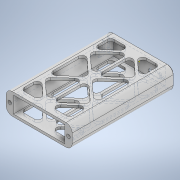
# Autodesk Inventor part: base
Saved by Autodesk Inventor 2021 (Build 250183000, 183)
## iProperties
Created: 2025-12-12
Part Number: base
Material: Generic
Document SubType Name: Modeling
Designer: Toby
Density: 1 g/cm^3
Appearance: Default
Author: Toby
Autodesk Inventor part; units mm, degrees
ref_plane "YZ Plane" through (0, 0, 0) normal (1, 0, 0) x (0, 1, 0)
ref_plane "XZ Plane" through (0, 0, 0) normal (0, 1, 0) x (-1, 0, 0)
ref_plane "XY Plane" through (0, 0, 0) normal (0, 0, 1) x (1, 0, 0)
sketch "Sketch1" plane through (0, 0, 0) normal (0, 0, 1) x (1, 0, 0)
  point P0 (0, 0)
sketch "Sketch2" plane through (0, 0, 0) normal (0, 0, 1) x (1, 0, 0)
  line L0 (-21, 6.75) -> (21, 6.75)
  line L1 (21, 6.75) -> (21, -6.75)
  line L2 (21, -6.75) -> (-21, -6.75)
  line L3 (-21, -6.75) -> (-21, 6.75)
  line L4 (-27, 8.75) -> (27, 8.75)
  line L5 (27, 8.75) -> (27, -8.75)
  line L6 (27, -8.75) -> (-27, -8.75)
  line L7 (-27, -8.75) -> (-27, 8.75)
  point P0 (0, 0)
  dimension "d0" = 42
  dimension "d1" = 13.5
  dimension "d2" = 2
  dimension "d3" = 2
  dimension "d4" = 6
  dimension "d5" = 6
  dimension "d6" = 6.75
  dimension "d7" = 21
  constraints: 16 end point, 4 parallel, 2 horizontal, 2 perpendicular
  measures "d0" distance of L0.start L0.end
  measures "d1" distance between parallel lines of L2 L0
  measures "d2" distance between parallel lines of L0 L4
  measures "d3" distance between parallel lines of L6 L2
  measures "d4" distance between parallel lines of L7 L3
  measures "d5" distance between parallel lines of L5 L1
  measures "d6" distance from line of point (0, 0) L0
  measures "d7" distance from line of point (0, 0) L3
extrude "Extrusion1" add sketch "Sketch2" along normal blind 82
sketch "Sketch3" plane through (0, 0, 0) normal (0, 0, -1) x (-1, 0, 0)
  line L0 (-27, -8.75) -> (-27, 8.75) projected
  line L1 (27, 8.75) -> (27, -8.75) projected
  line L2 (-27, 8.75) -> (27, 8.75)
  line L3 (27, 8.75) -> (27, -8.75)
  line L4 (27, -8.75) -> (-27, -8.75)
  line L5 (-27, -8.75) -> (-27, 8.75)
  point P0 (0, 0)
  constraints: 8 end point, 2 parallel, 1 horizontal, 1 perpendicular
extrude "Extrusion2" add sketch "Sketch3" along normal blind 1.2
fillet "Fillet1" radius 5 4 edges at (-27, 8.75, 40.4) (-27, -8.75, 40.4) (27, 8.75, 40.4) (27, -8.75, 40.4)
sketch "Sketch4" plane through (0, 0, 82) normal (0, 0, 1) x (1, 0, 0)
  line L0 (-21, -6.75) -> (-21, 6.75) projected
  line L1 (21, 6.75) -> (21, -6.75) projected
  line L2 (21, -6.75) -> (-21, -6.75) projected
  point P0 (0, 0)
  point P1 (-24, 0)
  point P2 (24, 0)
  dimension "d13" = 3
  dimension "d14" = 3
  dimension "d15" = 6.75
  dimension "d16" = 6.75
  measures "d13" distance from line of L0 point (-24, 0)
  measures "d14" distance from line of L1 point (24, 0)
  measures "d15" distance from line of L2 point (-24, 0)
  measures "d16" distance from line of L2 point (24, 0)
hole "Hole1" at (-24, 0, 82) at (24, 0, 82) direction (0, 0, -1) diameter 3 depth 8.8 tip angle 118
sketch "Sketch5" plane through (0, 0, 0) normal (0, 0, 1) x (1, 0, 0)
  line L0 (7.5, -1.05) -> (16.7, -1.05)
  line L1 (16.7, -1.05) -> (16.7, -4.55)
  line L2 (16.7, -4.55) -> (7.5, -4.55)
  line L3 (7.5, -4.55) -> (7.5, -1.05)
  line L4 (21, -6.75) -> (-21, -6.75) projected
  line L5 (21, 6.75) -> (21, -6.75) projected
  point P0 (0, 0)
  dimension "d24" = 2.2
  dimension "d25" = 3.5
  dimension "d26" = 9.2
  dimension "d27" = 4.3
  constraints: 8 end point, 2 parallel, 1 horizontal, 1 perpendicular
  measures "d24" distance between parallel lines of L4 L2
  measures "d25" distance between parallel lines of L2 L0
  measures "d26" distance of L0.start L0.end
  measures "d27" distance between parallel lines of L5 L1
extrude "Extrusion3" cut sketch "Sketch5" against normal blind 1.2
fillet "Fillet2" radius 1 4 edges at (16.7, -1.05, -0.6) (16.7, -4.55, -0.6) (7.5, -4.55, -0.6) (7.5, -1.05, -0.6)
sketch "Sketch6" plane through (0, 0, 0) normal (0, 0, 1) x (1, 0, 0)
  circle A0 centre (18.8, -2.8) radius 0.75
  line L0 (21, 6.75) -> (21, -6.75) projected
  line L1 (15.7, -4.55) -> (8.5, -4.55) projected
  line L2 (8.5, -1.05) -> (15.7, -1.05) projected
  point P0 (0, 0)
  dimension "d31" = 1.5
  dimension "d32" = 2.2
  dimension "d33" = 1.75
  dimension "d34" = 1.75
  constraints: 1 centre point
  measures "d31" diameter of A0
  measures "d32" distance from line of L0 A0.centre
  measures "d33" distance from line of L1 A0.centre
  measures "d34" distance from line of A0.centre L2
extrude "Extrusion4" cut sketch "Sketch6" against normal blind 1.2
chamfer "Chamfer1" distance 0.6 angle 45 8 edges at (12.1, -1.05, -1.2) (7.7929, -1.3429, -1.2) (7.5, -2.8, -1.2) (7.7929, -4.2571, -1.2) (12.1, -4.55, -1.2) (16.4071, -4.2571, -1.2) (16.7, -2.8, -1.2) (16.4071, -1.3429, -1.2)
chamfer "Chamfer2" distance 0.6 angle 45 8 edges at (0, 8.75, -1.2) (25.5355, 7.2855, -1.2) (27, 0, -1.2) (25.5355, -7.2855, -1.2) (0, -8.75, -1.2) (-25.5355, -7.2855, -1.2) (-27, 0, -1.2) (-25.5355, 7.2855, -1.2)
sketch "Sketch7" plane through (-22, 8.75, 82) normal (0, 1, 0) x (1, 0, 0)
  line L0 (2, 78.6) -> (42, 78.6)
  line L1 (42, 78.6) -> (42, 5)
  line L2 (42, 5) -> (2, 5)
  line L3 (2, 5) -> (2, 78.6)
  line L4 (0, 82.6) -> (44, 82.6) projected
  line L5 (0, 0) -> (0, 82.6) projected
  line L6 (44, 82.6) -> (44, 0) projected
  line L7 (44, 0) -> (0, 0) projected
  line L8 (44, 83.2) -> (48.4, 83.2) projected
  point P0 (22, 82)
  dimension "d43" = 4
  dimension "d44" = 2
  dimension "d45" = 2
  dimension "d46" = 5
  dimension "d47" = 4.6
  constraints: 8 end point, 2 parallel, 1 horizontal, 1 perpendicular
  measures "d43" distance between parallel lines of L0 L4
  measures "d44" distance between parallel lines of L5 L3
  measures "d45" distance between parallel lines of L6 L1
  measures "d46" distance between parallel lines of L7 L2
  measures "d47" distance between parallel lines of L0 L8
extrude "Extrusion5" cut sketch "Sketch7" against normal blind 30 contours L0 L1 L2 L3
sketch "Sketch8" plane through (-22, -8.75, 82) normal (0, -1, 0) x (1, 0, 0)
  line L0 (42, -5) -> (2, -5) projected
  line L1 (2, -78.6) -> (42, -78.6) projected
  line L2 (22, -5) -> (22, -78.6) construction
  line L3 (21, -5) -> (21, -78.6)
  line L4 (23, -78.6) -> (23, -5)
  arc A0 (23, -5) -> (21, -5) centre (22, -5) ccw
  arc A1 (21, -78.6) -> (23, -78.6) centre (22, -78.6) ccw
  line L5 (42, -78.6) -> (42, -5) projected
  line L6 (2, -5) -> (2, -78.6) projected
  line L7 (42, -23.4) -> (22, -5) construction
  line L8 (42.6771, -22.6641) -> (22.6771, -4.2641)
  line L9 (21.3229, -5.7359) -> (41.3229, -24.1359)
  arc A2 (41.3229, -24.1359) -> (42.6771, -22.6641) centre (42, -23.4) ccw
  arc A3 (22.6771, -4.2641) -> (21.3229, -5.7359) centre (22, -5) ccw
  line L10 (22, -5) -> (2, -23.4) construction
  line L11 (21.3229, -4.2641) -> (1.3229, -22.6641)
  line L12 (2.6771, -24.1359) -> (22.6771, -5.7359)
  arc A4 (22.6771, -5.7359) -> (21.3229, -4.2641) centre (22, -5) ccw
  arc A5 (1.3229, -22.6641) -> (2.6771, -24.1359) centre (2, -23.4) ccw
  line L13 (2, -23.4) -> (22, -41.8) construction
  arc A6 (2.6771, -22.6641) -> (1.3229, -24.1359) centre (2, -23.4) ccw
  arc A7 (21.3229, -42.5359) -> (22.6771, -41.0641) centre (22, -41.8) ccw
  line L14 (22, -41.8) -> (2, -60.2) construction
  line L15 (21.3229, -41.0641) -> (1.3229, -59.4641)
  line L16 (2.6771, -60.9359) -> (22.6771, -42.5359)
  arc A8 (22.6771, -42.5359) -> (21.3229, -41.0641) centre (22, -41.8) ccw
  arc A9 (1.3229, -59.4641) -> (2.6771, -60.9359) centre (2, -60.2) ccw
  line L17 (2, -60.2) -> (22, -78.6) construction
  line L18 (1.3229, -60.9359) -> (21.3229, -79.3359)
  line L19 (22.6771, -77.8641) -> (2.6771, -59.4641)
  arc A10 (2.6771, -59.4641) -> (1.3229, -60.9359) centre (2, -60.2) ccw
  arc A11 (21.3229, -79.3359) -> (22.6771, -77.8641) centre (22, -78.6) ccw
  line L20 (42, -23.4) -> (22, -41.8) construction
  line L21 (41.3229, -22.6641) -> (21.3229, -41.0641)
  line L22 (22.6771, -42.5359) -> (42.6771, -24.1359)
  arc A12 (42.6771, -24.1359) -> (41.3229, -22.6641) centre (42, -23.4) ccw
  arc A13 (21.3229, -41.0641) -> (22.6771, -42.5359) centre (22, -41.8) ccw
  line L23 (2, -23.4) -> (42, -60.2) construction
  line L24 (1.3229, -24.1359) -> (41.3229, -60.9359)
  line L25 (42.6771, -59.4641) -> (2.6771, -22.6641)
  arc A14 (2.6771, -22.6641) -> (1.3229, -24.1359) centre (2, -23.4) ccw
  arc A15 (41.3229, -60.9359) -> (42.6771, -59.4641) centre (42, -60.2) ccw
  line L26 (42, -60.2) -> (22, -78.6) construction
  line L27 (41.3229, -59.4641) -> (21.3229, -77.8641)
  line L28 (22.6771, -79.3359) -> (42.6771, -60.9359)
  arc A16 (42.6771, -60.9359) -> (41.3229, -59.4641) centre (42, -60.2) ccw
  arc A17 (21.3229, -77.8641) -> (22.6771, -79.3359) centre (22, -78.6) ccw
  point P0 (22, -82)
  point P1 (42, -41.8)
  point P2 (32, -14.2)
  point P3 (12, -14.2)
  point P4 (12, -32.6)
  point P5 (12, -51)
  point P6 (12, -69.4)
  point P7 (32, -32.6)
  point P8 (22, -41.8)
  point P9 (32, -69.4)
  point P10 (2, -22.4)
  point P11 (1.3229, -22.6641)
  point P12 (1.3229, -24.1359)
  point P13 (20.523, -41.8)
  point P14 (2, -58.8412)
  point P15 (2, -59.2)
  point P16 (1.3229, -59.4641)
  point P17 (1.3229, -60.9359)
  point P18 (23.477, -41.8)
  point P19 (22.6771, -4.2641)
  point P20 (20.523, -5)
  point P21 (2, -22.0412)
  point P22 (3.477, -23.4)
  point P23 (21, -7.2788)
  point P24 (21, -39.5212)
  point P25 (40.523, -23.4)
  point P26 (23, -39.5212)
  point P27 (23, -7.2788)
  point P28 (23, -44.0788)
  point P29 (40.523, -60.2)
  point P30 (23, -76.3212)
  point P31 (3.477, -60.2)
  point P32 (21, -44.0788)
  point P33 (21, -76.3212)
  dimension "d50" = 2
  dimension "d51" = 73.6
  dimension "d52" = 36.8
  dimension "d53" = 18.4
  dimension "d54" = 18.4
  dimension "d55" = 2
  dimension "d56" = 2
  dimension "d57" = 2
  dimension "d58" = 2
  dimension "d59" = 2
  dimension "d60" = 2
  dimension "d61" = 2
  dimension "d62" = 2
  constraints: 68 end point, 36 point on circle, 32 tangent, 18 centre point, 12 midpoint, 10 parallel, 4 point on line, 1 concentric, 1 perpendicular
  measures "d50" diameter of A1
  measures "d51" distance between parallel lines of L1 L0
  measures "d52" distance from line of point (42, -41.8) L0
  measures "d53" distance from line of L0 L7.start
  measures "d54" distance from line of L1 L23.end
  measures "d55" diameter of A3
  measures "d56" diameter of A5
  measures "d57" diameter of A7
  measures "d58" diameter of A9
  measures "d59" diameter of A11
  measures "d60" diameter of A13
  measures "d61" diameter of A15
  measures "d62" diameter of A17
extrude "Extrusion6" add sketch "Sketch8" against normal blind 2 contours A4 L12 L9 A3 L0 | A0 L8 L0 | L0 L8 L5 A12 L21 L9 L4 | L0 A0 | L4 L9 L12 A4 | L3 L12 L25 A6 L6 L11 L0 | A3 L9 L12 L3 | L4 L21 L25 L3 L12 L9 | L8 A12 L5 | L21 L9 A2 L5 L22 L25 L4 | L4 L25 L21 | L21 A12 L5 A2 L9 | L25 L21 L15 L3 | L3 L15 L24 L6 A5 L12 L25 | L12 A5 L6 A6 L25 | A12 A2 L5 | L25 L22 L4 | L4 A7 L25 | L25 A8 L21 | L6 A5 A6 | L15 A13 L3 | L3 L24 L15 | A2 L22 L5 | L4 L22 A7 | A7 A13 A8 | L25 L5 A16 L27 L24 L4 L22 | L6 L24 A5 | A13 L24 L3 | L24 L3 L16 L19 A10 L6 L15 | L4 L24 L16 L22 | L16 L24 A7 | L25 A16 L5 | L24 L16 L3 | L4 L27 L19 L3 L16 L24 | A16 A15 L5 | L5 A15 L24 L27 A16 | A10 L19 L16 A9 L6 | L6 A9 A10 | L27 L24 A15 L5 L28 L1 L4 | L4 A11 L19 L27 | A15 L28 L5 | L19 L27 A17 L3 | L3 L1 L18 L6 A9 L16 L19 | L6 L18 A9 | A1 L1 | L1 L28 A1 | L1 A17 L27 L19 A11 | A1 L18 L1
fillet "Fillet3" radius 3 30 edges at (20, -7.75, 77) (1.477, -7.75, 77) (1, -7.75, 74.7212) (-1, -7.75, 74.7212) (-1.477, -7.75, 77) (-20, -7.75, 77) (-20, -7.75, 59.9588) (-18.523, -7.75, 58.6) (-20, -7.75, 57.2412) (-1, -7.75, 42.4788) (-1.477, -7.75, 40.2) (-1, -7.75, 37.9212) (1, -7.75, 37.9212) (1.477, -7.75, 40.2) (1, -7.75, 42.4788) (18.523, -7.75, 58.6) (20, -7.75, 59.9588) (20, -7.75, 57.2412) (20, -7.75, 23.1588) (18.523, -7.75, 21.8) (20, -7.75, 20.4412) (20, -7.75, 3.4) (1.477, -7.75, 3.4) (1, -7.75, 5.6788) (-1, -7.75, 5.6788) (-1.477, -7.75, 3.4) (-20, -7.75, 3.4) (-20, -7.75, 20.4412) (-18.523, -7.75, 21.8) (-20, -7.75, 23.1588)
sketch "Sketch9" plane through (-22, 8.75, 82) normal (0, 1, 0) x (1, 0, 0)
  line L0 (2, 5) -> (42, 5) projected
  line L1 (2, 78.6) -> (42, 78.6) projected
  line L2 (42, 78.6) -> (42, 5) projected
  line L3 (2, 78.6) -> (2, 5) projected
  line L4 (22, 5) -> (22, 78.6) construction
  line L5 (23, 5) -> (23, 78.6)
  line L6 (21, 78.6) -> (21, 5)
  arc A0 (21, 5) -> (23, 5) centre (22, 5) ccw
  arc A1 (23, 78.6) -> (21, 78.6) centre (22, 78.6) ccw
  line L7 (42, 60.2) -> (2, 23.4) construction
  line L8 (41.3229, 60.9359) -> (1.3229, 24.1359)
  line L9 (2.6771, 22.6641) -> (42.6771, 59.4641)
  arc A2 (42.6771, 59.4641) -> (41.3229, 60.9359) centre (42, 60.2) ccw
  arc A3 (1.3229, 24.1359) -> (2.6771, 22.6641) centre (2, 23.4) ccw
  line L10 (42, 23.4) -> (2, 60.2) construction
  line L11 (42.6771, 24.1359) -> (2.6771, 60.9359)
  line L12 (1.3229, 59.4641) -> (41.3229, 22.6641)
  arc A4 (41.3229, 22.6641) -> (42.6771, 24.1359) centre (42, 23.4) ccw
  arc A5 (2.6771, 60.9359) -> (1.3229, 59.4641) centre (2, 60.2) ccw
  line L13 (42, 60.2) -> (22, 78.6) construction
  line L14 (42.6771, 60.9359) -> (22.6771, 79.3359)
  line L15 (21.3229, 77.8641) -> (41.3229, 59.4641)
  arc A6 (41.3229, 59.4641) -> (42.6771, 60.9359) centre (42, 60.2) ccw
  arc A7 (22.6771, 79.3359) -> (21.3229, 77.8641) centre (22, 78.6) ccw
  line L16 (2, 60.2) -> (22, 78.6) construction
  line L17 (2.6771, 59.4641) -> (22.6771, 77.8641)
  line L18 (21.3229, 79.3359) -> (1.3229, 60.9359)
  arc A8 (1.3229, 60.9359) -> (2.6771, 59.4641) centre (2, 60.2) ccw
  arc A9 (22.6771, 77.8641) -> (21.3229, 79.3359) centre (22, 78.6) ccw
  line L19 (42, 23.4) -> (22, 5) construction
  line L20 (41.3229, 24.1359) -> (21.3229, 5.7359)
  line L21 (22.6771, 4.2641) -> (42.6771, 22.6641)
  arc A10 (42.6771, 22.6641) -> (41.3229, 24.1359) centre (42, 23.4) ccw
  arc A11 (21.3229, 5.7359) -> (22.6771, 4.2641) centre (22, 5) ccw
  point P0 (22, 82)
  point P1 (22, 41.8)
  point P2 (22, 41.8)
  point P3 (22, 41.8)
  point P4 (22, 41.8)
  point P5 (32, 69.4)
  point P6 (12, 69.4)
  point P7 (32, 14.2)
  point P8 (23, 7.2788)
  point P9 (23, 39.5212)
  point P10 (40.523, 23.4)
  point P11 (21, 44.0788)
  point P12 (3.477, 60.2)
  point P13 (21, 76.3212)
  point P14 (40.523, 60.2)
  point P15 (23, 44.0788)
  point P16 (23, 76.3212)
  point P17 (20.523, 41.8)
  point P18 (21, 39.5212)
  point P19 (22.6771, 4.2641)
  point P20 (42.6771, 22.6641)
  point P21 (23.477, 41.8)
  point P22 (1.3229, 60.9359)
  dimension "d66" = 73.6
  dimension "d67" = 18.4
  dimension "d68" = 36.8
  dimension "d69" = 18.4
  dimension "d70" = 2
  dimension "d71" = 2
  dimension "d72" = 2
  dimension "d73" = 2
  dimension "d74" = 2
  dimension "d75" = 2
  constraints: 48 end point, 24 point on circle, 24 tangent, 12 centre point, 9 parallel, 8 midpoint, 3 concentric, 3 point on line, 1 perpendicular
  measures "d66" distance between parallel lines of L1 L0
  measures "d67" distance from line of L0 L10.start
  measures "d68" distance from line of L0 point (22, 41.8)
  measures "d69" distance from line of L1 L7.start
  measures "d70" diameter of A1
  measures "d71" diameter of A3
  measures "d72" diameter of A5
  measures "d73" diameter of A7
  measures "d74" diameter of A9
  measures "d75" diameter of A11
extrude "Extrusion7" add sketch "Sketch9" against normal blind 2 contours A11 L20 L5 L0 | L0 A0 | L6 L9 L12 L5 L20 A11 | A3 L8 L3 | L3 L8 L12 L6 L9 A3 | L5 L20 L12 A4 L2 L21 L0 | L0 L21 A0 | L6 L12 L9 | L12 L8 L6 | L6 L8 L11 L5 L9 L12 | L9 L5 L12 | L12 A8 L3 | L3 A8 L17 L11 L6 L8 L12 | L2 A4 L21 | L5 L9 L11 L2 A10 L20 L12 | L20 A10 L2 A4 L12 | L6 L11 L8 | L5 L11 L9 | A8 A5 L3 | L3 A5 L11 L17 A8 | L2 A10 A4 | L6 L17 L15 L5 L8 L11 | L8 L5 L11 | L5 L8 L15 A6 L2 L9 L11 | A5 L18 L3 | L3 L18 L1 L6 L17 L11 A5 | L2 L11 A10 | L6 A7 L15 L17 | L2 A6 L9 | A1 L1 | L1 L18 A1 | L1 A9 L17 L15 A7 | L17 A9 L5 L15 | L5 L1 L14 L2 A2 L8 L15 | L8 A2 L2 A6 L15 | L2 A2 A6 | A1 L14 L1 | L2 L14 A2
sketch "Sketch10" plane through (-22, 8.75, 82) normal (0, 1, 0) x (1, 0, 0)
  arc A0 (2, 22.4) -> (2.6771, 22.6641) centre (2, 23.4) ccw projected
  line L0 (22, 5) -> (2, 23.4) construction
  line L1 (22.6771, 5.7359) -> (2.6771, 24.1359)
  line L2 (1.3229, 22.6641) -> (21.3229, 4.2641)
  arc A1 (21.3229, 4.2641) -> (22.6771, 5.7359) centre (22, 5) ccw
  arc A2 (2.6771, 24.1359) -> (1.3229, 22.6641) centre (2, 23.4) ccw
  point P0 (22, 82)
  point P1 (12, 14.2)
  dimension "d78" = 2
  constraints: 8 end point, 4 point on circle, 4 tangent, 2 centre point, 1 coincident, 1 midpoint, 1 parallel
  measures "d78" diameter of A2
extrude "Extrusion8" add sketch "Sketch10" against normal blind 2
fillet "Fillet4" radius 3 30 edges at (20, 7.75, 77) (20, 7.75, 59.9588) (18.523, 7.75, 58.6) (20, 7.75, 57.2412) (1.477, 7.75, 77) (1, 7.75, 74.7212) (-1, 7.75, 74.7212) (-1.477, 7.75, 77) (-20, 7.75, 77) (-20, 7.75, 59.9588) (-18.523, 7.75, 58.6) (-20, 7.75, 57.2412) (-20, 7.75, 23.1588) (-18.523, 7.75, 21.8) (-20, 7.75, 20.4412) (-1.477, 7.75, 3.4) (-20, 7.75, 3.4) (1.477, 7.75, 3.4) (1, 7.75, 5.6788) (-1, 7.75, 5.6788) (20, 7.75, 3.4) (20, 7.75, 20.4412) (20, 7.75, 23.1588) (18.523, 7.75, 21.8) (1.477, 7.75, 40.2) (1, 7.75, 42.4788) (-1, 7.75, 42.4788) (-1.477, 7.75, 40.2) (-1, 7.75, 37.9212) (1, 7.75, 37.9212)
sketch "Sketch11" plane through (0, 0, -1.2) normal (0, 0, -1) x (-1, 0, 0)
  line L0 (27, 3.75) -> (22.4, 3.75)
  line L1 (22.4, 3.75) -> (22.4, -3.75)
  line L2 (22.4, -3.75) -> (27, -3.75)
  line L3 (27, -3.75) -> (27, 3.75)
  line L4 (27, -3.75) -> (26.4, -3.75) projected
  line L5 (27, 3.75) -> (26.4, 3.75) projected
  line L6 (27, -3.75) -> (27, 3.75) projected
  line L7 (21, -6.75) -> (21, 6.75) projected
  point P0 (0, 0)
  dimension "d82" = 4.6
  dimension "d83" = 1.4
  constraints: 8 end point, 3 collinear, 2 parallel, 1 horizontal, 1 perpendicular
  measures "d82" distance between parallel lines of L3 L1
  measures "d83" distance between parallel lines of L1 L7
extrude "Extrusion9" cut sketch "Sketch11" against normal blind 12
sketch "Sketch12" plane through (0, 0, -1.2) normal (0, 0, -1) x (-1, 0, 0)
  arc A0 (27, 3.75) -> (22, 8.75) centre (22, 3.75) ccw projected
  line L0 (26.4, -3.75) -> (22.4, -3.75) projected
  line L1 (27, 3.75) -> (25.5, 3.75)
  line L2 (25.5, 3.75) -> (25.5, -3.75)
  line L3 (25.5, -3.75) -> (27, -3.75)
  line L4 (27, -3.75) -> (27, 3.75)
  point P0 (0, 0)
  dimension "d86" = 1.5
  constraints: 8 end point, 2 parallel, 1 horizontal, 1 perpendicular, 1 point on circle, 1 point on line
  measures "d86" distance between parallel lines of L2 L4
extrude "Extrusion10" add sketch "Sketch12" against normal blind 4
chamfer "Chamfer3" distance 0.6 angle 45 1 edges at (-27, 0, -1.2)
fillet "Fillet5" radius 1 4 edges at (-24.7, 3.75, 10.8) (-24.7, -3.75, 10.8) (-26.25, 3.75, 2.8) (-26.25, -3.75, 2.8)
fillet "Fillet6" radius 0.6 9 edges at (-25.5, 3.75, 3.3) (-25.5, 3.75, 0.8) (-22.4, 3.4571, 10.5071) (-22.4, 0, 10.8) (-22.4, -3.4571, 10.5071) (-22.4, -3.75, 4.3) (-22.4, 3.75, 4.3) (-25.5, -3.75, 3.3) (-25.5, -3.75, 0.8)
body "Solid1"
